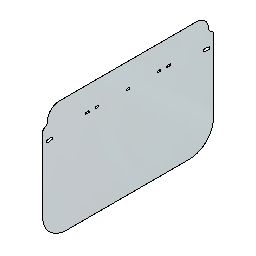
Dentist_shield (Autodesk Fusion 360 archive; units mm, degrees)
design "Dentist shield" references "Shield holes"
Autodesk Fusion 360 part; units mm, degrees
derive "ExternalDerived" from "Shield holes v11"
sketch "Sketch1" plane through (0, 0, 0) normal (1, 0, 0) x (0, 1, 0)
  line L0 (169.678, -26.6) -> (169.678, -23.4)
  line L1 (169.678, -23.4) -> (177.178, -23.4)
  line L2 (177.178, -26.6) -> (169.678, -26.6)
  line L3 (177.178, -23.4) -> (177.178, -26.6)
  line L4 (150.7435, -26.6) -> (150.7435, -23.4)
  line L5 (150.7435, -23.4) -> (155.7435, -23.4)
  line L6 (155.7435, -26.6) -> (150.7435, -26.6)
  line L7 (155.7435, -23.4) -> (155.7435, -26.6)
  line L8 (85.9655, -26.6) -> (85.9655, -23.4)
  line L9 (85.9655, -23.4) -> (91.4655, -23.4)
  line L10 (91.4655, -26.6) -> (85.9655, -26.6)
  line L11 (91.4655, -23.4) -> (91.4655, -26.6)
  line L12 (21.6875, -26.6) -> (21.6875, -23.4)
  line L13 (21.6875, -23.4) -> (26.6875, -23.4)
  line L14 (26.6875, -26.6) -> (21.6875, -26.6)
  line L15 (26.6875, -23.4) -> (26.6875, -26.6)
  line L16 (0.2529, -26.6) -> (0.2529, -23.4)
  line L17 (0.2529, -23.4) -> (7.7529, -23.4)
  line L18 (7.7529, -26.6) -> (0.2529, -26.6)
  line L19 (7.7529, -23.4) -> (7.7529, -26.6)
  line L20 (-88.7845, 25) -> (266.2155, 25)
  line L21 (266.2155, 25) -> (266.2155, -165)
  line L22 (216.2155, -215) -> (-38.7845, -215)
  line L23 (-88.7845, -165) -> (-88.7845, 25)
  line L24 (88.7155, 25) -> (88.7155, -215) construction
  line L25 (-88.7845, -25) -> (266.2155, -25) construction
  line L26 (-88.7845, -40) -> (266.2155, -40) construction
  line L27 (-80.2845, -38.6324) -> (-69.5001, -36.4655) construction
  line L28 (-69.5001, -36.4655) -> (-68.5151, -41.3676) construction
  line L29 (-68.5151, -41.3676) -> (-79.2995, -43.5345) construction
  line L30 (-79.2995, -43.5345) -> (-80.2845, -38.6324) construction
  line L31 (246.931, -36.4655) -> (257.7155, -38.6324) construction
  line L32 (257.7155, -38.6324) -> (256.7305, -43.5345) construction
  line L33 (256.7305, -43.5345) -> (245.9461, -41.3676) construction
  line L34 (245.9461, -41.3676) -> (246.931, -36.4655) construction
  line L35 (252.3233, -37.549) -> (251.3383, -42.451) construction
  line L36 (-74.8923, -37.549) -> (-73.9073, -42.451) construction
  line L37 (-80.2845, -38.6324) -> (-88.7845, -38.6324) construction
  line L38 (257.7155, -38.6324) -> (266.2155, -38.6324) construction
  arc A0 (-88.7845, -165) -> (-38.7845, -215) centre (-38.7845, -165) ccw
  arc A1 (216.2155, -215) -> (266.2155, -165) centre (216.2155, -165) ccw
  line L39 (-69.0076, -38.9165) -> (0.2529, -25) construction
  line L40 (177.178, -25) -> (246.4386, -38.9165) construction
  line L41 (-80.2845, -27.872) -> (-79.9514, -32.8609) construction
  line L42 (-79.9514, -32.8609) -> (-68.9758, -32.128) construction
  line L43 (-68.9758, -32.128) -> (-69.3089, -27.1391) construction
  line L44 (-69.3089, -27.1391) -> (-80.2845, -27.872) construction
  line L45 (-69.1424, -29.6336) -> (0.2529, -25) construction
  line L46 (-80.2845, -27.872) -> (-88.7845, -27.872) construction
  line L47 (-88.7845, -30) -> (266.2155, -30) construction
  line L48 (-74.7967, -27.5056) -> (-74.4636, -32.4944) construction
  line L49 (257.7155, -27.872) -> (246.7399, -27.1391) construction
  line L50 (252.2277, -27.5056) -> (251.8946, -32.4944) construction
  line L51 (246.7399, -27.1391) -> (246.4068, -32.128) construction
  line L52 (246.4068, -32.128) -> (257.3824, -32.8609) construction
  line L53 (257.3824, -32.8609) -> (257.7155, -27.872) construction
  line L54 (177.178, -25) -> (246.5734, -29.6336) construction
  line L55 (257.7155, -27.872) -> (266.2155, -27.872) construction
  line L56 (-68.7187, -36.7487) -> (-79.6216, -38.2072)
  line L57 (-79.6216, -38.2072) -> (-80.2845, -33.2513)
  line L58 (-80.2845, -33.2513) -> (-69.3816, -31.7928)
  line L59 (-69.3816, -31.7928) -> (-68.7187, -36.7487)
  line L60 (-74.8331, -32.5221) -> (-74.1701, -37.4779) construction
  line L61 (-69.0502, -34.2708) -> (0.2529, -25) construction
  line L62 (-80.2845, -33.2513) -> (-88.7845, -33.2513) construction
  line L63 (-88.7845, -35) -> (266.2155, -35) construction
  line L64 (257.0525, -38.2072) -> (257.7155, -33.2513)
  line L65 (246.8126, -31.7928) -> (246.1497, -36.7487)
  line L66 (257.7155, -33.2513) -> (246.8126, -31.7928)
  line L67 (246.1497, -36.7487) -> (257.0525, -38.2072)
  line L68 (246.4811, -34.2708) -> (177.178, -25) construction
  line L69 (257.7155, -33.2513) -> (266.2155, -33.2513) construction
  line L70 (252.2641, -32.5221) -> (251.6011, -37.4779) construction
  point P0 (88.7155, -25)
  point P1 (88.7155, -25)
  point P2 (-74.3998, -40)
  point P3 (251.8308, -40)
  point P4 (-74.6302, -30)
  point P5 (252.0612, -30)
  point P6 (-74.5016, -35)
  point P7 (251.998, -32.3294)
  point P8 (251.9326, -35)
  dimension "d4" = 15
  dimension "d5" = 11
  dimension "d6" = 5
  dimension "d7" = 8.5
  dimension "d8" = 240
  dimension "d9" = 355
  dimension "d10" = 50
  dimension "d12" = 50
  dimension "d15" = 5
  dimension "d19" = 10
  constraint horizontal L20
  constraint vertical L21
  constraint horizontal L22
  constraint vertical L23
  constraint coincident L23 L25.start
  constraint coincident L21 L25.end
  constraint perpendicular L21 L25
  constraint coincident L25 P1
  constraint coincident L24 P1
  constraint coincident P1 P0
  constraint coincident L23 L26.start
  constraint coincident L21 L26.end
  constraint perpendicular L21 L26
  constraint coincident L26 P2
  constraint equal L29 L31
  constraint equal L28 L32
  constraint midpoint L31 L35.start
  constraint midpoint L33 L35.end
  constraint midpoint L27 L36.start
  constraint midpoint L29 L36.end
  constraint midpoint P2 L36
  constraint midpoint L35 P3
  constraint coincident L26 P3
  constraint coincident L23 L37.end
  constraint horizontal L37
  constraint coincident L21 L38.end
  constraint perpendicular L21 L38
  constraint equal L37 L38
  constraint coincident L20 L24.start
  constraint coincident L22 L24.end
  constraint tangent L23 A0
  constraint tangent L22 A0
  constraint tangent L22 A1
  constraint tangent L21 A1
  constraint equal A0 A1
  constraint midpoint L25 P1
  constraint midpoint L28 L39.start
  constraint midpoint L16 L39.end
  constraint perpendicular L28 L39
  constraint perpendicular L28 L29
  constraint perpendicular L27 L28
  constraint perpendicular L29 L30
  constraint midpoint L3 L40.start
  constraint midpoint L34 L40.end
  constraint perpendicular L34 L40
  constraint perpendicular L33 L34
  constraint perpendicular L31 L34
  constraint perpendicular L31 L32
  constraint perpendicular L41 L42
  constraint perpendicular L42 L43
  constraint perpendicular L41 L44
  constraint midpoint L43 L45.start
  constraint coincident L23 L46.end
  constraint perpendicular L23 L46
  constraint equal L37 L46
  constraint equal L27 L42
  constraint equal L28 L41
  constraint coincident L23 L47.start
  constraint coincident L21 L47.end
  constraint perpendicular L21 L47
  constraint midpoint L44 L48.start
  constraint midpoint L42 L48.end
  constraint midpoint L48 P4
  constraint coincident L47 P4
  constraint perpendicular L43 L45
  constraint perpendicular L51 L52
  constraint perpendicular L52 L53
  constraint perpendicular L49 L51
  constraint midpoint L50.start L49
  constraint midpoint L50.end L52
  constraint midpoint P5 L50
  constraint midpoint L51 L54.end
  constraint perpendicular L51 L54
  constraint equal L31 L49
  constraint equal L34 L51
  constraint coincident L21 L55.end
  constraint perpendicular L21 L55
  constraint equal L38 L55
  constraint coincident L47 P5
  constraint midpoint L60.start L58
  constraint midpoint L60.end L56
  constraint horizontal L62
  constraint midpoint L61.start L59
  constraint perpendicular L59 L61
  constraint perpendicular L56 L59
  constraint perpendicular L58 L59
  constraint perpendicular L56 L57
  constraint equal L46 L62
  constraint coincident L39.end L45.end
  constraint coincident L23 L62.end
  constraint equal L43 L59
  constraint equal L44 L58
  constraint coincident L23 L63.start
  constraint coincident L21 L63.end
  constraint perpendicular L21 L63
  constraint midpoint L60 P6
  constraint coincident L63 P6
  constraint midpoint L68.start L65
  constraint perpendicular L65 L68
  constraint perpendicular L65 L67
  constraint perpendicular L65 L66
  constraint perpendicular L64 L67
  constraint coincident L40.start L54.start
  constraint equal L51 L64
  constraint equal L49 L66
  constraint coincident L21 L69.end
  constraint perpendicular L21 L69
  constraint equal L55 L69
  constraint midpoint L66 L70.start
  constraint midpoint L67 L70.end
  constraint midpoint L70 P8
  constraint coincident L63 P8
  constraint coincident L20.start L23.end
  constraint perpendicular L22 L24
  constraint coincident L20.end L21.start
  measures "d4" distance of L25.start L26.start
  measures "d5" distance of L27.start L27.end
  measures "d6" distance of L27.start L29.end
  measures "d7" distance of L27.start L37.end
  measures "d8" distance of L24.start L24.end
  measures "d9" distance of L26.start L26.end
  measures "d10" distance of L24.start P1
  measures "d12" radius of A0
  measures "d15" distance of L25.start L47.start
  measures "d19" distance of L25.start L63.start
extrude "Extrude1" add sketch "Sketch1" along normal blind 0.2
sketch "Sketch2" plane through (0, 0, 0) normal (1, 0, 0) x (0, 1, 0)
  line L0 (266.2155, 25) -> (-88.7845, 25) construction
  line L1 (-88.7845, 25) -> (-88.7845, -165) construction
  line L2 (266.2155, -165) -> (266.2155, 25) construction
  arc A0 (-83.7845, -7.5) -> (-88.7845, -15) centre (-80.6595, -15) ccw
  arc A1 (-83.7845, -7.5) -> (-78.7845, 0) centre (-86.9095, 0) ccw
  arc A2 (-53.7845, 25) -> (-78.7845, 0) centre (-53.7845, 0) ccw
  line L3 (-88.7845, -15) -> (266.2155, -15) construction
  line L4 (-86.9095, 0) -> (266.2155, 0) construction
  line L5 (256.2155, 25) -> (256.2155, -15) construction
  arc A3 (266.2155, -15) -> (261.2155, -7.5) centre (258.0905, -15) ccw
  arc A4 (256.2155, 0) -> (261.2155, -7.5) centre (264.3405, 0) ccw
  arc A5 (256.2155, 0) -> (231.2155, 25) centre (231.2155, 0) ccw
  line L6 (-53.7845, 25) -> (231.2155, 25)
  line L7 (-88.7845, -15) -> (-88.7845, 25)
  line L8 (-53.7845, 25) -> (-88.7845, 25)
  line L9 (231.2155, 25) -> (266.2155, 25)
  line L10 (266.2155, 25) -> (266.2155, -15)
  dimension "d22" = 15
  dimension "d23" = 25
  dimension "d24" = 25
  dimension "d25" = 10
  dimension "d26" = 10
  dimension "d27" = 25
  constraint tangent L1 A0
  constraint coincident L1 A0.end
  constraint tangent A0 A1
  constraint equal A0 A1
  constraint coincident A1.end A2.end
  constraint coincident L0 A2.start
  constraint tangent A1 A2
  constraint coincident L2 L3.end
  constraint perpendicular L2 L3
  constraint coincident A1.centre L4.start
  constraint coincident L2 L4.end
  constraint perpendicular L2 L4
  constraint coincident L0 L5.start
  constraint coincident L3 L5.end
  constraint perpendicular L3 L5
  constraint tangent L2 A3
  constraint tangent L5 A4
  constraint coincident L4 A4.start
  constraint coincident L5 A4.start
  constraint tangent A3 A4
  constraint equal A3 A4
  constraint tangent L0 A5
  constraint coincident L0 A5.end
  constraint coincident L0.end L1.start
  constraint tangent A2 L8
  constraint coincident L0.start L2.end
  measures "d22" vertical distance of A1.end A0.end
  measures "d23" radius of A2
  measures "d24" distance of L0 A1.end
  measures "d25" horizontal distance of A1.end A0.end
  measures "d26" distance of L3.end L5.end
  measures "d27" radius of A5
extrude "Extrude2" cut sketch "Sketch2" along normal blind 0.2

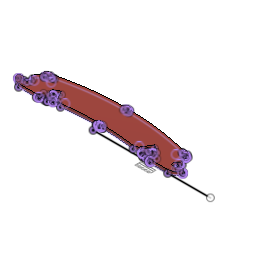
design "top_piece"
Autodesk Fusion 360 part; units mm, degrees
sketch "Main body" plane through (0, 0, 0) normal (0, 0, 1) x (1, 0, 0)
  line L0 (0, 0) -> (0, 30.7494) construction
  line L1 (60, 23.4426) -> (-60, 23.4426) construction
  line L2 (-70, 13.4426) -> (70, 13.4426) construction
  line L3 (-70, 13.4426) -> (-70, 0) construction
  line L4 (70, 0) -> (70, 13.4426) construction
  line L5 (-77.5, 7.9426) -> (77.5, 7.9426) construction
  circle A0 centre (-70, 7.9426) radius 2.9426 construction
  arc A1 (-77.8598, 6.7985) -> (-70, 0) centre (-70, 7.9426) ccw
  line L6 (-76.8702, 7.9426) -> (-72.9426, 7.9426)
  arc A2 (-76.8702, 7.9426) -> (-77.8598, 6.7985) centre (-76.8702, 6.9426) ccw
  circle A3 centre (70, 7.9426) radius 2.9426 construction
  line L7 (72.9426, 7.9426) -> (76.8702, 7.9426)
  arc A4 (70, 0) -> (77.8598, 6.7985) centre (70, 7.9426) ccw
  arc A5 (77.8598, 6.7985) -> (76.8702, 7.9426) centre (76.8702, 6.9426) ccw
  arc A6 (-72.9426, 7.9426) -> (-68.8487, 10.6506) centre (-70, 7.9426) ccw
  arc A7 (68.8487, 10.6506) -> (72.9426, 7.9426) centre (70, 7.9426) ccw
  line L8 (-77.5, 30.7494) -> (77.5, 30.7494) construction
  line L9 (77.5, 30.7494) -> (77.5, 0) construction
  line L10 (77.5, 0) -> (-77.5, 0) construction
  line L11 (-77.5, 0) -> (-77.5, 30.7494) construction
  line L12 (-60, 23.4426) -> (-60, 13.4426) construction
  line L13 (60, 23.4426) -> (60, 13.4426) construction
  line L14 (-70, 0) -> (70, 0)
  arc A8 (59.6571, 23.5271) -> (-59.6571, 23.5271) centre (0, -219.2506) ccw
  arc A9 (-60.3719, 23.2864) -> (-70, 13.4426) centre (-53.134, 6.5765) ccw
  arc A10 (-70, 13.4426) -> (-68.8487, 10.6506) centre (-68.0067, 12.6311) ccw
  line L15 (-60, 13.4426) -> (-66.0104, 19.453) construction
  arc A11 (70, 13.4426) -> (60.3719, 23.2864) centre (53.134, 6.5765) ccw
  line L16 (66.0105, 19.4529) -> (60, 13.4426) construction
  arc A12 (68.8487, 10.6506) -> (70, 13.4426) centre (68.0067, 12.6311) ccw
  arc A13 (-59.6571, 23.5271) -> (-60.3719, 23.2864) centre (-58.5833, 19.1571) ccw
  arc A14 (60.3719, 23.2864) -> (59.6571, 23.5271) centre (58.5833, 19.1571) ccw
  point P0 (0, 13.4426)
  point P1 (0, 7.9426)
  point P2 (70, 7.9426)
  point P3 (-72.9426, 7.9426)
  point P4 (72.9426, 7.9426)
  point P5 (-77.5, 7.9426)
  point P6 (-77.5, 13.4426)
  point P7 (-77.5, 23.4426)
  point P8 (-70, 0)
  point P9 (0, 30.7494)
  point P10 (-70, 30.7494)
  point P11 (-60, 30.7494)
  point P12 (0, 30.2837)
  point P13 (-66.6872, 16.948)
  point P14 (-66.0104, 19.453)
  dimension "d450" = 5.8852
  dimension "d456" = 1
  dimension "d457" = 5.8852
  dimension "d458" = 1
  dimension "d459" = 7.9426
  dimension "d460" = 5.5
  dimension "d461" = 10
  dimension "d463" = 70
  dimension "d465" = 7.5
  dimension "d467" = 10
  dimension "d520" = 250
  dimension "d551" = 8.5
  dimension "d552" = 8.5
  dimension "d561" = 4.5
  dimension "d562" = 4.5
  dimension "d572" = 2.1521
  dimension "d573" = 2.1521
  dimension "d574" = 10
  constraint coincident L0.start origin
  constraint vertical L0
  constraint perpendicular L0 L1
  constraint horizontal L2
  constraint coincident L2 P0
  constraint midpoint L2 P0
  constraint coincident L0 P0
  constraint perpendicular L2 L3
  constraint perpendicular L4 L5
  constraint coincident L5 P1
  constraint midpoint L5 P1
  constraint coincident L0 P1
  constraint coincident L5 A0.centre
  constraint coincident L3 A0.centre
  constraint coincident L5 P2
  constraint coincident L4 P2
  constraint coincident A0.centre A1.centre
  constraint coincident L5 L6.start
  constraint coincident L5 P3
  constraint parallel L5 L6
  constraint coincident A0 P3
  constraint coincident P3 L6.end
  constraint coincident A1.start A2.end
  constraint tangent L6 A2
  constraint tangent A1 A2
  constraint coincident P2 A3.centre
  constraint coincident L5 P4
  constraint coincident L5 L7.end
  constraint parallel L5 L7
  constraint coincident A3 P4
  constraint coincident P4 L7.start
  constraint tangent L5 A5
  constraint tangent A4 A5
  constraint coincident A0 A6.end
  constraint horizontal L8
  constraint vertical L9
  constraint horizontal L10
  constraint vertical L11
  constraint coincident L11 P5
  constraint coincident L11 P6
  constraint coincident L11 P7
  constraint coincident L10 P8
  constraint midpoint L0.start L10
  constraint coincident L5 P5
  constraint coincident L2 P6
  constraint coincident L1 P7
  constraint midpoint L8 P9
  constraint coincident L8 P10
  constraint coincident L3 P10
  constraint coincident P5 L5.start
  constraint coincident L3 P8
  constraint coincident P9 L0.end
  constraint coincident L2 L12.end
  constraint perpendicular L2 L12
  constraint coincident L2 L13.end
  constraint perpendicular L2 L13
  constraint coincident L8 P11
  constraint coincident L12 P11
  constraint coincident A1 P8
  constraint coincident L4.start L10
  constraint coincident P8 L3.end
  constraint perpendicular L0 L5
  constraint coincident L0 P12
  constraint tangent A9 A10
  constraint tangent A0 A10
  constraint coincident P14 L15.end
  constraint tangent A11 A12
  constraint tangent A7 A12
  constraint coincident P9 A8
  constraint coincident A9 P14
  constraint coincident L1.end A8
  constraint coincident L1.end A9
  constraint tangent A8 A13
  constraint tangent A9 A13
  constraint coincident A11 L16.start
  constraint coincident L1.start A8
  constraint coincident L1.start A11
  constraint tangent A8 A14
  constraint tangent A11 A14
  measures "d450" diameter of A0
  measures "d456" radius of A2
  measures "d457" diameter of A3
  measures "d458" radius of A5
  measures "d459" distance of L10.end P5
  measures "d460" distance of P5 P6
  measures "d461" distance of P6 P7
  measures "d463" distance of P9 P10
  measures "d465" distance of L8.start P10
  measures "d467" distance of P10 P11
  measures "d520" radius of A8
  measures "d551" distance of L12.end P14
  measures "d552" distance of L13.end L16.start
  measures "d561" radius of A13
  measures "d562" radius of A14
  measures "d572" radius of A12
  measures "d573" radius of A10
  measures "d574" distance of L2.end L13.end
sketch "Inner connectors _ old" plane through (0, 0, 0) normal (0, 0, 1) x (1, 0, 0)
  line L0 (-77.5, 7.9426) -> (77.5, 7.9426) construction
  line L1 (77.5, 0) -> (-77.5, 0) construction
  line L2 (-77.5, 0) -> (77.5, 0) construction
  line L3 (-35.4314, 0) -> (-43.4022, 13.8057)
  line L4 (-37.9718, 0) -> (-42.5574, 7.9426) construction
  line L5 (-43.5574, 7.9426) -> (-42.5574, 7.9426) construction
  line L6 (-40.6522, 9.0426) -> (-42.5574, 7.9426) construction
  arc A0 (-45.5, 5.1751) -> (-43.5574, 7.9426) centre (-46.5, 7.9426) ccw
  arc A1 (-46.5, 0) -> (-40.3845, 2.8745) centre (-46.5, 7.9426) ccw
  line L7 (-46.5, 7.9426) -> (-46.5, 0) construction
  arc A2 (-40.3845, 2.8745) -> (-40.2884, 4.0126) centre (-41.1545, 3.5126) ccw
  line L8 (-46.5, 0) -> (-35.4314, 0)
  line L9 (35.6624, 0) -> (43.5754, 13.7057)
  line L10 (37.9718, 0) -> (42.5574, 7.9426) construction
  line L11 (43.5574, 7.9426) -> (42.5574, 7.9426) construction
  line L12 (42.5574, 7.9426) -> (40.8254, 8.9426) construction
  arc A3 (43.5574, 7.9426) -> (45.5, 5.1751) centre (46.5, 7.9426) ccw
  arc A4 (40.3845, 2.8745) -> (46.5, 0) centre (46.5, 7.9426) ccw
  arc A5 (40.2884, 4.0126) -> (40.3845, 2.8745) centre (41.1545, 3.5126) ccw
  line L13 (46.5, 7.9426) -> (46.5, 0) construction
  line L14 (35.6624, 0) -> (46.5, 0)
  line L15 (-47.5, 5.1751) -> (-45.5, 5.1751)
  line L16 (-40.2884, 4.0126) -> (-42.0574, 7.0766)
  arc A6 (-42.0574, 7.0766) -> (-43.5574, 7.9426) centre (-43.5574, 6.2105) ccw
  line L17 (40.2884, 4.0126) -> (42.0574, 7.0766)
  arc A7 (43.5574, 7.9426) -> (42.0574, 7.0766) centre (43.5574, 6.2105) ccw
  line L18 (47.5, 5.1751) -> (45.5, 5.1751)
  line L19 (43.5754, 13.7057) -> (47.3852, 11.5061)
  arc A8 (-49.4426, 7.9426) -> (-47.5, 5.1751) centre (-46.5, 7.9426) ccw
  line L20 (-43.4022, 13.8057) -> (-47.3852, 11.5061)
  arc A9 (-47.3852, 11.5061) -> (-49.4426, 7.9426) centre (-45.3277, 7.9426) ccw
  arc A10 (47.5, 5.1751) -> (49.4426, 7.9426) centre (46.5, 7.9426) ccw
  arc A11 (49.4426, 7.9426) -> (47.3852, 11.5061) centre (45.3277, 7.9426) ccw
  point P0 (-70, 7.9426)
  point P1 (70, 7.9426)
  point P2 (-46.5, 5.1751)
  point P3 (46.5, 5.1751)
  point P4 (-43.4022, 13.8057)
  dimension "d469" = 23.5
  dimension "d471" = 23.5
  dimension "d486" = 60
  dimension "d487" = 2.2
  dimension "d488" = 1
  dimension "d492" = 1
  dimension "d493" = 60
  dimension "d495" = 1
  dimension "d498" = 2
  dimension "d500" = 1
  dimension "d571" = 5
  dimension "d575" = 2.9426
  dimension "d577" = 1
  dimension "d578" = 1
  dimension "d579" = 2.9426
  dimension "d585" = 5
  constraint coincident L1.end L2.start
  constraint coincident L1.start L2.end
  constraint coincident L1 L3.start
  constraint coincident L1 L4.start
  constraint parallel L3 L4
  constraint coincident L0 L5.start
  constraint parallel L0 L5
  constraint coincident L3 L6.start
  constraint perpendicular L3 L6
  constraint coincident L2 A1.start
  constraint coincident A0.centre A1.centre
  constraint vertical L7
  constraint tangent A1 A2
  constraint coincident L4 A2.end
  constraint coincident L2 L9.start
  constraint coincident L2 L10.start
  constraint parallel L9 L10
  constraint coincident L0 L11.start
  constraint parallel L0 L11
  constraint perpendicular L10 L12
  constraint coincident L9 L12.end
  constraint coincident L2 A4.end
  constraint coincident A3.centre A4.centre
  constraint coincident L10 A5.start
  constraint tangent L10 A5
  constraint tangent A4 A5
  constraint coincident L1 A4.end
  constraint perpendicular L1 L13
  constraint coincident A0 L15.end
  constraint horizontal L15
  constraint coincident L4 L16.end
  constraint tangent A2 L16
  constraint parallel L4 L16
  constraint tangent L16 A6
  constraint coincident L10 L17.end
  constraint parallel L10 L17
  constraint tangent L17 A7
  constraint tangent L0 A6
  constraint tangent L0 A7
  constraint coincident A3 L18.end
  constraint horizontal L18
  constraint perpendicular L9 L19
  constraint coincident A0.start L15.end
  constraint coincident L0 A0.centre
  constraint midpoint L15 P2
  constraint coincident L7 P2
  constraint coincident L0 A3.centre
  constraint midpoint L18 P3
  constraint coincident L13 P3
  constraint coincident A3.end L18.end
  constraint coincident P4 L3.end
  constraint coincident L0 A8.start
  constraint coincident A8.start A9.end
  constraint coincident L20.end A9.start
  constraint tangent A8 A9
  constraint tangent L20 A9
  constraint perpendicular L3 L20
  constraint tangent A10 A11
  constraint tangent L19 A11
  constraint coincident L0 A10.end
  measures "d469" distance of P0 A0.centre
  measures "d471" distance of P1 A3.centre
  measures "d486" angle of L2 L3
  measures "d487" distance of L3 L4
  measures "d488" distance of L5.start L4.end
  measures "d492" radius of A2
  measures "d493" angle of L2 L10
  measures "d495" distance of L11.start L10.end
  measures "d498" distance of L10.end L12.end
  measures "d500" radius of A5
  measures "d571" distance of L11.start L19
  measures "d575" radius of A0
  measures "d577" distance of L15.start P2
  measures "d578" distance of L13 A3.end
  measures "d579" radius of A3
  measures "d585" distance of L5.start L20
sketch "Inner curve" plane through (0, 0, 0) normal (0, 0, 1) x (1, 0, 0)
  line L0 (-70, 0) -> (70, 0) construction
  line L1 (0, 30.7494) -> (0, 0) construction
  arc A0 (59.6571, 23.5271) -> (-59.6571, 23.5271) centre (0, -219.2506) ccw
  arc A1 (53.3069, 0) -> (-53.3069, 0) centre (0, -244.2506) ccw
  line L2 (-70, 0) -> (70, 0) construction
  line L3 (-53.3069, 0) -> (53.3069, 0)
  point P0 (0, 30.7494)
  point P1 (0, 5.7494)
  dimension "d505" = 25
  dimension "d586" = 250
  constraint coincident P0 L1.start
  constraint coincident L1.end origin
  constraint coincident L1 P1
  constraint coincident L0 A1.start
  constraint coincident L0 A1.end
  constraint midpoint P1 A1
  constraint coincident L0.start L2.start
  constraint coincident L0.end L2.end
  measures "d505" distance of P0 P1
  measures "d586" radius of A1
sketch "Spike top" plane through (0, 0, 0) normal (0, 0, 1) x (1, 0, 0)
  arc A0 (-1, 33.2494) -> (-2.5, 31.7494) centre (-1, 31.7494) ccw
  line L0 (2.5, 31.7494) -> (2.5, 30.7369)
  line L1 (-1, 33.2494) -> (1, 33.2494)
  arc A1 (2.5, 31.7494) -> (1, 33.2494) centre (1, 31.7494) ccw
  line L2 (-2.5, 30.7369) -> (-2.5, 31.7494)
  line L3 (0, 0) -> (0, 33.2494) construction
  arc A2 (59.6571, 23.5271) -> (-59.6571, 23.5271) centre (0, -219.2506) ccw
  point P0 (2.5, 33.2494)
  point P1 (-2.5, 33.2494)
  point P2 (0, 30.7494)
  dimension "d196" = 5
  dimension "d198" = 1.5
  dimension "d199" = 1.5
  dimension "d522" = 2.5
  constraint vertical L2
  constraint perpendicular L1 L2
  constraint vertical L0
  constraint coincident P1 L2
  constraint coincident P1 L1
  constraint tangent A0 L2
  constraint tangent A0 L1
  constraint coincident P0 L1
  constraint coincident P0 L0
  constraint tangent L1 A1
  constraint tangent L0 A1
  constraint coincident L3.start origin
  constraint vertical L3
  constraint midpoint L1 L3.end
  constraint coincident L2.start A2
  constraint coincident L0.end A2
  constraint coincident P2 A2
  measures "d196" distance of P0 P1
  measures "d198" radius of A0
  measures "d199" radius of A1
  measures "d522" distance of L3.end P2
sketch "Spike side" plane through (0, 0, 0) normal (0, 0, 1) x (1, 0, 0)
  line L0 (-64.6665, 23.7784) -> (-63.2744, 21.7019) construction
  line L1 (-66.8617, 22.3068) -> (-62.4714, 25.2501) construction
  line L2 (-66.8617, 22.3068) -> (-68.0588, 21.5042) construction
  line L3 (-62.4714, 25.2501) -> (-61.2782, 22.8639) construction
  line L4 (-68.0588, 21.5042) -> (-66.0092, 19.4542) construction
  arc A0 (-61.4625, 23.2324) -> (-64.3452, 23.9939) centre (-63.2391, 22.344) ccw
  arc A1 (-66.5432, 22.5203) -> (-66.7687, 20.2138) centre (-65.7079, 21.2744) ccw
  line L5 (-66.5432, 22.5203) -> (-64.3452, 23.9939)
  line L6 (-61.4625, 23.2324) -> (-61.2782, 22.8639)
  line L7 (-66.4461, 19.8912) -> (-61.4625, 23.2324) construction
  line L8 (-65.6155, 20.4481) -> (-65.3622, 20.0701)
  line L9 (-65.6155, 20.4481) -> (-66.4461, 19.8912)
  line L10 (-66.7687, 20.2138) -> (-66.4461, 19.8912)
  line L11 (66.8617, 22.3068) -> (62.4714, 25.2501) construction
  line L12 (66.4461, 19.8912) -> (61.4625, 23.2324) construction
  line L13 (66.8617, 22.3068) -> (68.0588, 21.5042) construction
  line L14 (64.6665, 23.7784) -> (63.2744, 21.7019) construction
  line L15 (62.4714, 25.2501) -> (61.2782, 22.8639) construction
  line L16 (65.6155, 20.4481) -> (66.4461, 19.8912)
  arc A2 (66.5432, 22.5203) -> (66.7687, 20.2138) centre (65.7079, 21.2744) cw
  line L17 (66.5432, 22.5203) -> (64.3452, 23.9939)
  line L18 (65.6155, 20.4481) -> (65.3622, 20.0701)
  arc A3 (61.4625, 23.2324) -> (64.3452, 23.9939) centre (63.2391, 22.344) cw
  line L19 (61.4625, 23.2324) -> (61.2782, 22.8639)
  line L20 (68.0588, 21.5042) -> (66.0092, 19.4542) construction
  line L21 (66.7687, 20.2138) -> (66.4461, 19.8912)
  arc A4 (-60.3719, 23.2864) -> (-70, 13.4426) centre (-53.134, 6.5765) ccw
  arc A5 (70, 13.4426) -> (60.3719, 23.2864) centre (53.134, 6.5765) ccw
  point P0 (0, 47.6931)
  point P1 (0, 45.6174)
  point P2 (-53.134, 6.5765)
  point P3 (-66.0104, 19.453)
  point P4 (53.134, 6.5765)
  point P5 (66.0105, 19.4529)
  dimension "d314" = 2.5
  dimension "d321" = 1.5
  dimension "d323" = 2.5
  dimension "d327" = 1.5
  dimension "d553" = 0.455
  dimension "d554" = 0.455
  dimension "d555" = 5
  dimension "d556" = 1
  dimension "d557" = 5
  dimension "d558" = 1
  dimension "d559" = 1
  dimension "d560" = 1
  constraint midpoint L0.start L1
  constraint perpendicular L0 L1
  constraint collinear L1 L2
  constraint tangent L1 A0
  constraint coincident L3 A0.start
  constraint coincident L1 A0.end
  constraint tangent L3 A0
  constraint coincident L4 A1.end
  constraint coincident L1 A1.start
  constraint tangent L1 A1
  constraint tangent L4 A1
  constraint coincident L4 L7.start
  constraint coincident L7 L8.start
  constraint perpendicular L7 L8
  constraint coincident L1.start L8
  constraint midpoint L14.start L11
  constraint perpendicular L11 L14
  constraint collinear L11 L13
  constraint tangent L11 A3
  constraint coincident L12.end L15
  constraint coincident L17.end L11
  constraint tangent L15 A3
  constraint coincident A2.end L20
  constraint coincident A2.start L11
  constraint tangent L11 A2
  constraint tangent A2 L20
  constraint coincident L12.start L20
  constraint coincident L16.start L12
  constraint perpendicular L12 L18
  constraint coincident L11.start L18
  constraint perpendicular L0 L7
  constraint coincident L12.end L19
  constraint perpendicular L12 L14
  constraint coincident L3.end A4
  constraint coincident L0.end A4
  constraint coincident L4.end A4
  constraint coincident L0 P2
  constraint coincident L14 P4
  constraint coincident L18.end A5
  constraint coincident L20.end A5
  constraint coincident L14.end A5
  constraint coincident L15 P4
  constraint coincident L20 P4
  constraint coincident L4 P2
  constraint coincident L3 P2
  constraint coincident L8.end A4
  constraint coincident A5 L15.end
  measures "d314" distance of L0.start L0.end
  measures "d321" radius of A1
  measures "d323" distance of L14.end L14.start
  measures "d327" radius of A2
  measures "d553" distance of L8.start L8.end
  measures "d554" distance of L18.end L16.start
  measures "d555" distance of A0.start L8.start
  measures "d556" distance of L7.start L8.start
  measures "d557" distance of L12.end L16.start
  measures "d558" distance of L12.start L16.start
  measures "d559" distance of L3.end A4.start
  measures "d560" distance of A5.end L15.end
sketch "Inner connector" plane through (0, 0, 0) normal (0, 0, 1) x (1, 0, 0)
  arc A0 (53.3069, 0) -> (-53.3069, 0) centre (0, -244.2506) ccw
  line L0 (-70, 7.9426) -> (-46.5, 7.9426) construction
  line L1 (-46.5, 9.3414) -> (-46.5, 1.3868) construction
  arc A1 (-45.5, 6.574) -> (-43.9516, 7.8702) centre (-46.5, 9.3414) ccw
  line L2 (-45.5, 6.574) -> (-47.5, 6.574)
  arc A2 (-49.0888, 7.9426) -> (-47.5, 6.574) centre (-46.5, 9.3414) ccw
  line L3 (-39.1005, 5.8677) -> (-43.6804, 13.8003)
  line L4 (-46.5, 9.3414) -> (-51.6932, 0.3466) construction
  line L5 (-43.6804, 13.8003) -> (-48.1631, 11.2121)
  line L6 (-46.5, 9.3414) -> (-43.9516, 7.8702) construction
  line L7 (-43.9516, 7.8702) -> (-43.0856, 8.3702)
  line L8 (-45.5, 6.574) -> (-45.5, 1.574) construction
  line L9 (-47.5, 6.574) -> (-47.5, 1.574) construction
  line L10 (-47.5, 1.574) -> (-45.5, 1.574)
  arc A3 (-45.5, 1.574) -> (-41.2154, 3.5616) centre (-46.5, 9.3414) ccw
  arc A4 (-50.4158, 2.5591) -> (-47.5, 1.574) centre (-46.5, 9.3414) ccw
  line L11 (-50.4158, 2.5591) -> (-51.4705, 0.7323)
  arc A5 (-52.128, 0.2543) -> (-51.4705, 0.7323) centre (-52.3365, 1.2323) ccw
  arc A6 (-48.1631, 11.2121) -> (-49.0888, 7.9426) centre (-46.9444, 9.1013) ccw
  line L12 (-43.0856, 8.3702) -> (-41.0242, 4.7996)
  arc A7 (-41.2154, 3.5616) -> (-41.0242, 4.7996) centre (-41.8902, 4.2996) ccw
  arc A8 (-39.1005, 5.8677) -> (-34.0886, 3.4144) centre (-34.7704, 8.3677) ccw
  line L13 (0, 0) -> (0, 5.7494)
  arc A9 (51.4705, 0.7323) -> (52.128, 0.2543) centre (52.3365, 1.2323) ccw
  line L14 (50.4158, 2.5591) -> (51.4705, 0.7323)
  arc A10 (47.5, 1.574) -> (50.4158, 2.5591) centre (46.5, 9.3414) ccw
  line L15 (47.5, 1.574) -> (45.5, 1.574)
  arc A11 (41.2154, 3.5616) -> (45.5, 1.574) centre (46.5, 9.3414) ccw
  arc A12 (41.0242, 4.7996) -> (41.2154, 3.5616) centre (41.8902, 4.2996) ccw
  line L16 (43.0856, 8.3702) -> (41.0242, 4.7996)
  line L17 (43.9516, 7.8702) -> (43.0856, 8.3702)
  arc A13 (43.9516, 7.8702) -> (45.5, 6.574) centre (46.5, 9.3414) ccw
  line L18 (45.5, 6.574) -> (47.5, 6.574)
  arc A14 (47.5, 6.574) -> (49.0888, 7.9426) centre (46.5, 9.3414) ccw
  arc A15 (49.0888, 7.9426) -> (48.1631, 11.2121) centre (46.9444, 9.1013) ccw
  line L19 (43.6804, 13.8003) -> (48.1631, 11.2121)
  line L20 (39.1005, 5.8677) -> (43.6804, 13.8003)
  arc A16 (34.0886, 3.4144) -> (39.1005, 5.8677) centre (34.7704, 8.3677) ccw
  point P0 (-70, 7.9426)
  point P1 (-46.5, 6.574)
  point P2 (-45.5, 6.574)
  dimension "d598" = 23.5
  dimension "d617" = 2.9426
  dimension "d618" = 2
  dimension "d620" = 1
  dimension "d623" = 30
  dimension "d624" = 5
  dimension "d625" = 60
  dimension "d633" = 30
  dimension "d634" = 2.2
  dimension "d635" = 1
  dimension "d636" = 1
  dimension "d637" = 5
  dimension "d638" = 5
  dimension "d639" = 23.5
  constraint coincident P0 L0.start
  constraint coincident L0.end L1
  constraint coincident A0 L1.end
  constraint vertical L1
  constraint horizontal L0
  constraint coincident L1 A1.centre
  constraint perpendicular L1 L2
  constraint midpoint L2 P1
  constraint coincident L1 P1
  constraint coincident P2 A1.start
  constraint coincident L1.start A1.centre
  constraint coincident A0 L4.end
  constraint perpendicular L3 L5
  constraint coincident A0 L8.end
  constraint perpendicular L2 L8
  constraint perpendicular L2 L9
  constraint horizontal L10
  constraint coincident L4 L11.end
  constraint parallel L4 L11
  constraint coincident A0 A5.start
  constraint tangent A0 A5
  constraint tangent L11 A5
  constraint tangent L5 A6
  constraint tangent A2 A6
  constraint coincident L0 A2.start
  constraint perpendicular L7 L12
  constraint parallel L3 L12
  constraint tangent L12 A7
  constraint tangent A3 A7
  constraint tangent L3 A8
  constraint coincident A0 A8.end
  constraint tangent A0 A8
  constraint coincident L13.start origin
  constraint midpoint A0 L13.end
  constraint symmetric P2 L13 A13.end
  constraint symmetric A1.end L13 L17.start
  constraint symmetric A1 L13 A13
  constraint symmetric L2.end L13 L18.end
  constraint symmetric A2.start L13 A14.end
  constraint symmetric A2 L13 A14
  constraint symmetric L3.start L13 L20.start
  constraint symmetric L3.end L13 L19.start
  constraint symmetric L5.end L13 A15.end
  constraint symmetric L7.end L13 L16.start
  constraint symmetric L8.end L13 L15.end
  constraint symmetric L9.end L13 A10.start
  constraint symmetric A3.end L13 A11.start
  constraint symmetric A3 L13 A11
  constraint symmetric A4.start L13 L14.start
  constraint symmetric A4 L13 A10
  constraint symmetric L11.end L13 A9.start
  constraint symmetric A5.start L13 A9.end
  constraint symmetric A5 L13 A9
  constraint symmetric A6 L13 A15
  constraint symmetric L12.end L13 A12.start
  constraint symmetric A7 L13 A12
  constraint symmetric A8.end L13 A16.start
  constraint symmetric A8 L13 A16
  measures "d598" distance of P0 L0.end
  measures "d617" radius of A1
  measures "d618" distance of P2 L2.end
  measures "d620" distance of A1.end L7.end
  measures "d623" angle of L1 L4
  measures "d624" distance of A1.end L5
  measures "d625" angle of L1 L6
  measures "d633" angle of L1 L3
  measures "d634" distance of L3 L7.end
  measures "d635" radius of A7
  measures "d636" radius of A5
  measures "d637" radius of A8
  measures "d638" distance of P2 L8.end
  measures "d639" distance of P0 L0.end
extrude "Extrude6" add sketch "Spike top" sketch "Main body" sketch "Spike side" along normal blind 3 of sketch 2 of sketch 3 makes body 1
extrude "Extrude7" cut sketch "Inner connector" sketch "Inner curve" along normal blind 3 contours A0 A11 A12 L16 L17 A13 L18 A14 A15 L19 L20 A16 | A0 A9 L14 A10 L15 | A0 A1 L2 A2 L3 L5 L7 A3 A6 L12 A7 A8 | A0 L10 A4 L11 A5 of sketch 2 bodies 1
copy_body "CopyPasteBodies6" bodies 1 makes body 2
move_body "Move9" bodies 2 to x (1, 0, 0) y (0, 1, 0) z (0, 0, 1) at (0, -25.45, 0)
sketch "Cutouts" plane through (0, 0, 0) normal (0, 0, 1) x (1, 0, 0)
  line L0 (-70, 0) -> (70, 0)
  arc A0 (-1, 7.7994) -> (-2.5, 6.2994) centre (-1, 6.2994) ccw construction
  line L1 (-2.5, 6.2994) -> (-2.5, 5.2869) construction
  line L2 (1, 7.7994) -> (-1, 7.7994) construction
  arc A1 (2.5, 6.2994) -> (1, 7.7994) centre (1, 6.2994) ccw construction
  line L3 (2.5, 5.2869) -> (2.5, 6.2994) construction
  line L4 (2.95, 5.2869) -> (2.95, 6.2994)
  arc A2 (2.95, 6.2994) -> (1, 8.2494) centre (1, 6.2994) ccw
  line L5 (1, 8.2494) -> (-1, 8.2494)
  arc A3 (-1, 8.2494) -> (-2.95, 6.2994) centre (-1, 6.2994) ccw
  line L6 (-2.95, 6.2994) -> (-2.95, 5.2869)
  line L7 (-2.95, 5.2869) -> (-2.95, 0)
  line L8 (2.95, 5.2869) -> (2.95, 0)
  dimension "d527" = 0.45
  constraint coincident L0 L7.end
  constraint perpendicular L0 L7
  constraint coincident L0 L8.end
  constraint perpendicular L0 L8
extrude "Extrude8" cut sketch "Cutouts" along normal blind 3 bodies 1
delete_body "RemoveBody3" bodies 2
sketch "Without inner connectors" plane through (0, 0, 0) normal (0, 0, 1) x (1, 0, 0)
  line L0 (2.95, 6.2994) -> (2.95, 5.732)
  line L1 (53.3069, 0) -> (70, 0)
  arc A0 (70, 0) -> (77.8598, 6.7985) centre (70, 7.9426) ccw
  arc A1 (77.8598, 6.7985) -> (76.8702, 7.9426) centre (76.8702, 6.9426) ccw
  line L2 (76.8702, 7.9426) -> (72.9426, 7.9426)
  arc A2 (68.8487, 10.6506) -> (72.9426, 7.9426) centre (70, 7.9426) ccw
  arc A3 (68.8487, 10.6506) -> (70, 13.4426) centre (68.0067, 12.6311) ccw
  arc A4 (70, 13.4426) -> (65.3622, 20.0701) centre (53.134, 6.5765) ccw
  line L3 (65.3622, 20.0701) -> (65.6155, 20.4481)
  line L4 (65.6155, 20.4481) -> (66.4461, 19.8912)
  line L5 (66.4461, 19.8912) -> (66.7687, 20.2138)
  arc A5 (66.7687, 20.2138) -> (66.5432, 22.5203) centre (65.7079, 21.2744) ccw
  line L6 (66.5432, 22.5203) -> (64.3452, 23.9939)
  arc A6 (64.3452, 23.9939) -> (61.4625, 23.2324) centre (63.2391, 22.344) ccw
  line L7 (61.4625, 23.2324) -> (61.2782, 22.8639)
  arc A7 (61.2782, 22.8639) -> (60.3719, 23.2864) centre (53.134, 6.5765) ccw
  arc A8 (60.3719, 23.2864) -> (59.6571, 23.5271) centre (58.5833, 19.1571) ccw
  arc A9 (59.6571, 23.5271) -> (2.5, 30.7369) centre (0, -219.2506) ccw
  line L8 (2.5, 30.7369) -> (2.5, 31.7494)
  arc A10 (2.5, 31.7494) -> (1, 33.2494) centre (1, 31.7494) ccw
  line L9 (1, 33.2494) -> (-1, 33.2494)
  arc A11 (-1, 33.2494) -> (-2.5, 31.7494) centre (-1, 31.7494) ccw
  line L10 (-2.5, 31.7494) -> (-2.5, 30.7369)
  arc A12 (-2.5, 30.7369) -> (-59.6571, 23.5271) centre (0, -219.2506) ccw
  arc A13 (-59.6571, 23.5271) -> (-60.3719, 23.2864) centre (-58.5833, 19.1571) ccw
  arc A14 (-60.3719, 23.2864) -> (-61.2782, 22.8639) centre (-53.134, 6.5765) ccw
  line L11 (-61.2782, 22.8639) -> (-61.4625, 23.2324)
  arc A15 (-61.4625, 23.2324) -> (-64.3452, 23.9939) centre (-63.2391, 22.344) ccw
  line L12 (-64.3452, 23.9939) -> (-66.5432, 22.5203)
  arc A16 (-66.5432, 22.5203) -> (-66.7687, 20.2138) centre (-65.7079, 21.2744) ccw
  line L13 (-66.7687, 20.2138) -> (-66.4461, 19.8912)
  line L14 (-66.4461, 19.8912) -> (-65.6155, 20.4481)
  line L15 (-65.6155, 20.4481) -> (-65.3622, 20.0701)
  arc A17 (-65.3622, 20.0701) -> (-70, 13.4426) centre (-53.134, 6.5765) ccw
  arc A18 (-70, 13.4426) -> (-68.8487, 10.6506) centre (-68.0067, 12.6311) ccw
  arc A19 (-72.9426, 7.9426) -> (-68.8487, 10.6506) centre (-70, 7.9426) ccw
  line L16 (-72.9426, 7.9426) -> (-76.8702, 7.9426)
  arc A20 (-76.8702, 7.9426) -> (-77.8598, 6.7985) centre (-76.8702, 6.9426) ccw
  arc A21 (-77.8598, 6.7985) -> (-70, 0) centre (-70, 7.9426) ccw
  line L17 (-70, 0) -> (-53.3069, 0)
  line L18 (-2.95, 5.732) -> (-2.95, 6.2994)
  arc A22 (-1, 8.2494) -> (-2.95, 6.2994) centre (-1, 6.2994) ccw
  line L19 (-1, 8.2494) -> (1, 8.2494)
  arc A23 (2.95, 6.2994) -> (1, 8.2494) centre (1, 6.2994) ccw
  arc A24 (41.3805, 2.3009) -> (36.4767, 3.0739) centre (0, -244.2506) ccw
  arc A25 (-36.4767, 3.0739) -> (-41.0722, 2.3524) centre (0, -244.2506) ccw
  arc A26 (53.3069, 0) -> (2.95, 5.732) centre (0, -244.2506) ccw
  arc A27 (-2.95, 5.732) -> (-53.3069, 0) centre (0, -244.2506) ccw
  dimension "d592" = 250
  dimension "d593" = 250
  measures "d592" radius of A24
  measures "d593" radius of A25
sketch "Inner connectors isolated" plane through (0, 0, 0) normal (0, 0, 1) x (1, 0, 0)
  arc A0 (-36.4767, 3.0739) -> (-41.0722, 2.3524) centre (0, -244.2506) ccw
  arc A1 (41.3805, 2.3009) -> (36.4767, 3.0739) centre (0, -244.2506) ccw
  arc A2 (53.3069, 0) -> (2.95, 5.732) centre (0, -244.2506) ccw
  arc A3 (-2.95, 5.732) -> (-53.3069, 0) centre (0, -244.2506) ccw
  dimension "d594" = 250
  dimension "d595" = 250
  measures "d594" radius of A0
  measures "d595" radius of A1
sketch "Sketch52" plane through (0, 0, 0) normal (0, 0, 1) x (1, 0, 0)
  line L0 (0, 0) -> (110, 0)
  line L1 (2.95, 6.2994) -> (2.95, 5.732)
  arc A0 (34.0886, 3.4144) -> (2.95, 5.732) centre (0, -244.2506) ccw
  arc A1 (34.0886, 3.4144) -> (39.1005, 5.8677) centre (34.7704, 8.3677) ccw
  line L2 (39.1005, 5.8677) -> (43.6804, 13.8003)
  line L3 (43.6804, 13.8003) -> (48.1631, 11.2121)
  arc A2 (49.0888, 7.9426) -> (48.1631, 11.2121) centre (46.9444, 9.1013) ccw
  arc A3 (47.5, 6.574) -> (49.0888, 7.9426) centre (46.5, 9.3414) ccw
  line L4 (47.5, 6.574) -> (45.5, 6.574)
  arc A4 (43.9516, 7.8702) -> (45.5, 6.574) centre (46.5, 9.3414) ccw
  line L5 (43.9516, 7.8702) -> (43.0856, 8.3702)
  line L6 (43.0856, 8.3702) -> (41.0242, 4.7996)
  arc A5 (41.0242, 4.7996) -> (41.2154, 3.5616) centre (41.8902, 4.2996) ccw
  arc A6 (41.2154, 3.5616) -> (44.679, 1.7245) centre (46.5, 9.3414) ccw
  arc A7 (45.5, 1.574) -> (44.679, 1.7245) centre (0, -244.2506) ccw
  line L7 (45.5, 1.574) -> (47.5, 1.574)
  arc A8 (47.5, 1.574) -> (50.4158, 2.5591) centre (46.5, 9.3414) ccw
  line L8 (50.4158, 2.5591) -> (51.4705, 0.7323)
  arc A9 (51.4705, 0.7323) -> (52.128, 0.2543) centre (52.3365, 1.2323) ccw
  arc A10 (53.3069, 0) -> (52.128, 0.2543) centre (0, -244.2506) ccw
  line L9 (53.3069, 0) -> (70, 0)
  arc A11 (70, 0) -> (77.8598, 6.7985) centre (70, 7.9426) ccw
  arc A12 (77.8598, 6.7985) -> (76.8702, 7.9426) centre (76.8702, 6.9426) ccw
  line L10 (76.8702, 7.9426) -> (72.9426, 7.9426)
  arc A13 (68.8487, 10.6506) -> (72.9426, 7.9426) centre (70, 7.9426) ccw
  arc A14 (68.8487, 10.6506) -> (70, 13.4426) centre (68.0067, 12.6311) ccw
  arc A15 (70, 13.4426) -> (65.3622, 20.0701) centre (53.134, 6.5765) ccw
  line L11 (65.3622, 20.0701) -> (65.6155, 20.4481)
  line L12 (65.6155, 20.4481) -> (66.4461, 19.8912)
  line L13 (66.4461, 19.8912) -> (66.7687, 20.2138)
  arc A16 (66.7687, 20.2138) -> (66.5432, 22.5203) centre (65.7079, 21.2744) ccw
  line L14 (66.5432, 22.5203) -> (64.3452, 23.9939)
  arc A17 (64.3452, 23.9939) -> (61.4625, 23.2324) centre (63.2391, 22.344) ccw
  line L15 (61.4625, 23.2324) -> (61.2782, 22.8639)
  arc A18 (61.2782, 22.8639) -> (60.3719, 23.2864) centre (53.134, 6.5765) ccw
  arc A19 (60.3719, 23.2864) -> (59.6571, 23.5271) centre (58.5833, 19.1571) ccw
  arc A20 (59.6571, 23.5271) -> (2.5, 30.7369) centre (0, -219.2506) ccw
  line L16 (2.5, 30.7369) -> (2.5, 31.7494)
  arc A21 (2.5, 31.7494) -> (1, 33.2494) centre (1, 31.7494) ccw
  line L17 (1, 33.2494) -> (-1, 33.2494)
  arc A22 (-1, 33.2494) -> (-2.5, 31.7494) centre (-1, 31.7494) ccw
  line L18 (-2.5, 31.7494) -> (-2.5, 30.7369)
  arc A23 (-2.5, 30.7369) -> (-59.6571, 23.5271) centre (0, -219.2506) ccw
  arc A24 (-59.6571, 23.5271) -> (-60.3719, 23.2864) centre (-58.5833, 19.1571) ccw
  arc A25 (-60.3719, 23.2864) -> (-61.2782, 22.8639) centre (-53.134, 6.5765) ccw
  line L19 (-61.2782, 22.8639) -> (-61.4625, 23.2324)
  arc A26 (-61.4625, 23.2324) -> (-64.3452, 23.9939) centre (-63.2391, 22.344) ccw
  line L20 (-64.3452, 23.9939) -> (-66.5432, 22.5203)
  arc A27 (-66.5432, 22.5203) -> (-66.7687, 20.2138) centre (-65.7079, 21.2744) ccw
  line L21 (-66.7687, 20.2138) -> (-66.4461, 19.8912)
  line L22 (-66.4461, 19.8912) -> (-65.6155, 20.4481)
  line L23 (-65.6155, 20.4481) -> (-65.3622, 20.0701)
  arc A28 (-65.3622, 20.0701) -> (-70, 13.4426) centre (-53.134, 6.5765) ccw
  arc A29 (-70, 13.4426) -> (-68.8487, 10.6506) centre (-68.0067, 12.6311) ccw
  arc A30 (-72.9426, 7.9426) -> (-68.8487, 10.6506) centre (-70, 7.9426) ccw
  line L24 (-72.9426, 7.9426) -> (-76.8702, 7.9426)
  arc A31 (-76.8702, 7.9426) -> (-77.8598, 6.7985) centre (-76.8702, 6.9426) ccw
  arc A32 (-77.8598, 6.7985) -> (-70, 0) centre (-70, 7.9426) ccw
  line L25 (-70, 0) -> (-53.3069, 0)
  arc A33 (-52.128, 0.2543) -> (-53.3069, 0) centre (0, -244.2506) ccw
  arc A34 (-52.128, 0.2543) -> (-51.4705, 0.7323) centre (-52.3365, 1.2323) ccw
  line L26 (-51.4705, 0.7323) -> (-50.4158, 2.5591)
  arc A35 (-50.4158, 2.5591) -> (-47.5, 1.574) centre (-46.5, 9.3414) ccw
  line L27 (-47.5, 1.574) -> (-45.5, 1.574)
  arc A36 (-44.679, 1.7245) -> (-45.5, 1.574) centre (0, -244.2506) ccw
  arc A37 (-44.679, 1.7245) -> (-41.2154, 3.5616) centre (-46.5, 9.3414) ccw
  arc A38 (-41.2154, 3.5616) -> (-41.0242, 4.7996) centre (-41.8902, 4.2996) ccw
  line L28 (-41.0242, 4.7996) -> (-43.0856, 8.3702)
  line L29 (-43.0856, 8.3702) -> (-43.9516, 7.8702)
  arc A39 (-45.5, 6.574) -> (-43.9516, 7.8702) centre (-46.5, 9.3414) ccw
  line L30 (-45.5, 6.574) -> (-47.5, 6.574)
  arc A40 (-49.0888, 7.9426) -> (-47.5, 6.574) centre (-46.5, 9.3414) ccw
  arc A41 (-48.1631, 11.2121) -> (-49.0888, 7.9426) centre (-46.9444, 9.1013) ccw
  line L31 (-48.1631, 11.2121) -> (-43.6804, 13.8003)
  line L32 (-43.6804, 13.8003) -> (-39.1005, 5.8677)
  arc A42 (-39.1005, 5.8677) -> (-34.0886, 3.4144) centre (-34.7704, 8.3677) ccw
  arc A43 (-2.95, 5.732) -> (-34.0886, 3.4144) centre (0, -244.2506) ccw
  line L33 (-2.95, 5.732) -> (-2.95, 6.2994)
  arc A44 (-1, 8.2494) -> (-2.95, 6.2994) centre (-1, 6.2994) ccw
  line L34 (-1, 8.2494) -> (1, 8.2494)
  arc A45 (2.95, 6.2994) -> (1, 8.2494) centre (1, 6.2994) ccw
  constraint coincident L0.start origin
  constraint horizontal L0
equation "spike_depth = 2,5 mm"
equation "spike_fillet = 1,5 mm"
equation "spike_width = 5 mm"
equation "shield_thickness = 0,2 mm"
equation "bitragion_breath = 160 mm"
equation "d196 = spike_width"
equation "d198 = spike_fillet"
equation "d199 = spike_fillet"
equation "d314 = spike_depth"
equation "d321 = spike_fillet"
equation "d323 = spike_depth"
equation "d327 = spike_fillet"
equation "kerf = 0,45 mm"
equation "d450 = connection_circle_diameter"
equation "d457 = connection_circle_diameter"
equation "d459 = connector_height * 1 mm + ( connection_circle_diameter / 2 )"
equation "d463 = ( 140 / 2 ) * 1 mm"
equation "min_circle_diameter = ( sqrt(connector_height ^ 2 + connector_width ^ 2) ) * 1 mm"
equation "connector_width = 2"
equation "connector_height = 5"
equation "connection_circle_diameter = min_circle_diameter + 0,5 mm"
equation "d487 = connector_width * 1,1 mm"
equation "d522 = spike_depth"
equation "d527 = kerf"
equation "shield_slot_depth = 0,455 mm"
equation "d553 = shield_slot_depth"
equation "d554 = shield_slot_depth"
equation "d571 = connector_height * 1 mm"
equation "d575 = connection_circle_diameter / 2"
equation "d577 = connector_width * 1 mm / 2"
equation "d578 = connector_width * 0,5 mm"
equation "d579 = connection_circle_diameter / 2"
equation "d617 = connection_circle_diameter / 2"
equation "d618 = connector_width * 1 mm"
equation "d624 = connector_height * 1 mm"
equation "d634 = connector_width * 1,1 mm"
